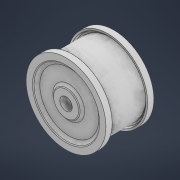
# Autodesk Inventor part: Tłok
Saved by Autodesk Inventor 2022 (Build 260153000, 153)
## iProperties
Created: 2023-04-12
Part Number: Tłok
Material: Ogólny
Document SubType Name: Modeling
Designer: jacek
Density: 1 g/cm^3
Appearance: Domyślna
Author: jacek
Autodesk Inventor part; units mm, degrees
ref_plane "YZ Plane" through (0, 0, 0) normal (1, 0, 0) x (0, 1, 0)
ref_plane "XZ Plane" through (0, 0, 0) normal (0, 1, 0) x (-1, 0, 0)
ref_plane "XY Plane" through (0, 0, 0) normal (0, 0, 1) x (1, 0, 0)
sketch "Szkic1" plane through (0, 0, 0) normal (1, 0, 0) x (0, 1, 0)
  line L0 (0, 0) -> (0, -54)
  line L1 (29, -10.5) -> (29, -43.5)
  line L2 (9, -39.9) -> (9, -14.1)
  line L3 (26.561, -8.5488) -> (10.561, -12.1488)
  line L4 (26.561, -45.4512) -> (10.561, -41.8512)
  arc A0 (29, -10.5) -> (26.561, -8.5488) centre (27, -10.5) ccw
  arc A1 (26.561, -45.4512) -> (29, -43.5) centre (27, -43.5) ccw
  arc A2 (9, -39.9) -> (10.561, -41.8512) centre (11, -39.9) ccw
  arc A3 (10.561, -12.1488) -> (9, -14.1) centre (11, -14.1) ccw
  line L5 (0, 0) -> (8, 0)
  line L6 (0, -54) -> (7.127, -54)
  line L7 (38, 0) -> (30.8902, 0)
  line L8 (38, -54) -> (30.8902, -54)
  arc A4 (26.2471, -3.607) -> (29.914, -0.7831) centre (26.3902, 0) ccw
  arc A5 (29.914, -53.2169) -> (26.2471, -50.393) centre (26.3902, -54) ccw
  arc A6 (8.0953, -0.75) -> (10.8811, -2.9976) centre (11, 0) ccw
  arc A7 (10.8811, -51.0024) -> (8.0953, -53.25) centre (11, -54) ccw
  line L9 (26.2471, -3.607) -> (10.8811, -2.9976)
  line L10 (26.2471, -50.393) -> (10.8811, -51.0024)
  line L11 (38, 0) -> (30, 0)
  line L12 (7.127, 0) -> (0, 0)
  line L13 (0, -54) -> (8, -54)
  line L14 (30, -54) -> (38, -54)
  arc A8 (30.8902, 0) -> (29.914, -0.7831) centre (30.8902, -1) ccw
  arc A9 (8.0953, -0.75) -> (7.127, 0) centre (7.127, -1) ccw
  arc A10 (7.127, -54) -> (8.0953, -53.25) centre (7.127, -53) ccw
  arc A11 (29.914, -53.2169) -> (30.8902, -54) centre (30.8902, -53) ccw
  line L15 (0, 0) -> (-7, 0)
  line L16 (-7, 0) -> (-7, -70)
  line L17 (33, -4) -> (35, -4)
  line L18 (35, -50) -> (33, -50)
  line L19 (33, -50) -> (33, -4)
  line L20 (38, 0) -> (38, -7)
  line L21 (38, -54) -> (38, -47)
  line L22 (38, -7) -> (36, -7)
  line L23 (36, -7) -> (35, -4)
  line L24 (38, -47) -> (36, -47)
  line L25 (36, -47) -> (35, -50)
  line L26 (38, -54) -> (38, -47)
  line L27 (38, -7) -> (38, 0)
  point P0 (9, -41.5)
  point P1 (9, -12.5)
  point P2 (9, -41.2105)
  point P3 (34, -27)
  dimension "d1" = 54
  dimension "d2" = 38
  dimension "d7" = 2
  dimension "d8" = 8
  dimension "d9" = 8
  dimension "d10" = 8
  dimension "d11" = 6
  dimension "d12" = 1
  dimension "d13" = 7
  dimension "d14" = 70
  dimension "d16" = 2
  dimension "d17" = 46
  dimension "d18" = 7
  dimension "d19" = 7
  dimension "d20" = 2
  dimension "d21" = 2
  constraints: 56 end point, 28 point on circle, 20 tangent, 12 centre point, 11 perpendicular, 11 point on line, 6 equal radius, 3 horizontal, 3 parallel, 3 vertical, 1 coincident
  measures "d1" distance of L0.start L0.end
  measures "d2" distance of L0.end L8.start
  measures "d7" radius of A0
  measures "d8" distance of L0.start L5.end
  measures "d9" distance of L11.end L7.start
  measures "d10" distance of L14.start L8.start
  measures "d11" diameter of A7
  measures "d12" radius of A8
  measures "d13" distance of L0.start L15.end
  measures "d14" distance of L15.end L16.end
  measures "d16" distance of L18.start L18.end
  measures "d17" distance of L17.end L18.start
  measures "d18" distance of L7.start L20.end
  measures "d19" distance of L8.start L21.end
  measures "d20" distance of L20.end L22.end
  measures "d21" distance of L21.end L24.end
revolve "Obrót2" add sketch "Szkic1" angle 360 about axis through (0, -7, 0) along (0, 0, -1)
